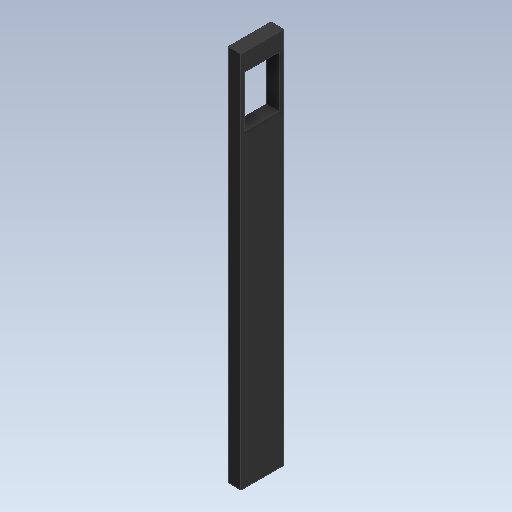
# Autodesk Inventor part: blade
Saved by Autodesk Inventor 2020 (Build 240168000, 168)
## iProperties
Created: 2021-07-04
Part Number: blade
Material: Rubber, Silicone
Document SubType Name: Modeling
Designer: pc
Density: 1.25 g/cm^3
Appearance: Rubber - Black
Mass: 752.781 g
Surface Area: 917.74 cm^2
Volume: 602.225 cm^3
Author: pc
Autodesk Inventor part; units mm, degrees
ref_plane "YZ Plane" through (0, 0, 0) normal (1, 0, 0) x (0, 1, 0)
ref_plane "XZ Plane" through (0, 0, 0) normal (0, 1, 0) x (-1, 0, 0)
ref_plane "XY Plane" through (0, 0, 0) normal (0, 0, 1) x (1, 0, 0)
sketch "Sketch1" plane through (0, 0, 0) normal (1, 0, 0) x (0, 1, 0)
  line L0 (10.4573, 9.6454) -> (-548.3427, 9.6454)
  line L1 (-548.3427, 9.6454) -> (-548.3427, -53.8546)
  line L2 (-548.3427, -53.8546) -> (10.4573, -53.8546)
  line L3 (10.4573, -53.8546) -> (10.4573, 9.6454)
  point P0 (0, 0)
  dimension "d0" = 558.8
  dimension "d1" = 63.5
  constraints: 8 end point, 2 parallel, 1 horizontal, 1 perpendicular
  measures "d0" distance of L2.end L1.end
  measures "d1" distance of L1.end L0.end
extrude "Extrusion1" add sketch "Sketch1" along normal blind 19.05
sketch "Sketch2" plane through (19.05, 0, 0) normal (1, 0, 0) x (0, 0, -1)
  line L0 (-4.0419, -15.157) -> (46.7581, -15.157)
  line L1 (46.7581, -15.157) -> (46.7581, -91.357)
  line L2 (46.7581, -91.357) -> (-4.0419, -91.357)
  line L3 (-4.0419, -91.357) -> (-4.0419, -15.157)
  point P0 (0, 0)
  dimension "d4" = 50.8
  dimension "d5" = 76.2
  constraints: 8 end point, 2 parallel, 1 horizontal, 1 perpendicular
  measures "d4" distance of L1.end L2.end
  measures "d5" distance of L0.end L1.end
extrude "Extrusion2" cut sketch "Sketch2" against normal blind 19.05
body "Solid1"
